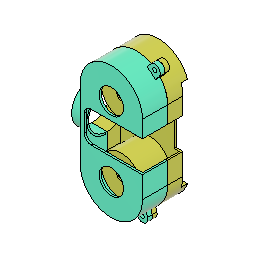
Nerf Ultra 2 cage v5 (Autodesk Fusion 360 design; units mm, degrees)
Autodesk Fusion 360 part; units mm, degrees
note: some values were not read from the file. Set by a fixed rule: which sketch regions a step uses.
sketch "Sketch1" plane through (0, 0, 0) normal (0, 0, 1) x (1, 0, 0)
  line L0 (23, 48.75) -> (-23, 48.75)
  line L1 (-23, 48.75) -> (-23, -48.75)
  line L2 (-23, -48.75) -> (23, -48.75)
  line L3 (23, -48.75) -> (23, 48.75)
  line L4 (23, 48.75) -> (-23, -48.75) construction
  line L5 (-23, 48.75) -> (23, -48.75) construction
  arc A0 (23, 25.75) -> (-23, 25.75) centre (0, 25.75) ccw
  arc A1 (-23, -25.75) -> (23, -25.75) centre (0, -25.75) ccw
  dimension "d1" = 46
  dimension "d2" = 97.5
  constraint perpendicular L0 L1
  constraint parallel L0 L2
  constraint parallel L1 L3
  constraint horizontal L0
  constraint coincident L4 origin
  constraint coincident L5 origin
  constraint tangent L3 A0
  constraint coincident L3 A0.start
  constraint coincident L1 A0.end
  constraint tangent L0 A0
  constraint tangent L1 A0
  constraint coincident L3 A1.end
  constraint coincident L1 A1.start
  constraint tangent L2 A1
  constraint tangent L3 A1
  constraint tangent L1 A1
  measures "d1" distance of L1.end L2.end
  measures "d2" distance of L0.end L1.end
  measures "d34" distance of L0.start
  measures "d93" diameter of L0.start
extrude "Extrude1" add sketch "Sketch1" along normal blind 16 contours L1 L3 A0 A1 makes body 1
sketch "Sketch2" plane through (0, 0, 16) normal (0, 0, 1) x (1, 0, 0)
  arc A0 (-23, -25.75) -> (23, -25.75) centre (0, -25.75) ccw
  line L0 (23, -25.75) -> (23, 25.75)
  arc A1 (23, 25.75) -> (-23, 25.75) centre (0, 25.75) ccw
  line L1 (-23, 25.75) -> (-23, -25.75)
  line L2 (0, 0) -> (-28, 0) construction
  line L3 (-23, 25) -> (-33, 25)
  line L4 (-33, 25) -> (-33, -25)
  line L5 (-33, -25) -> (-23, -25)
  line L6 (-23, -25) -> (-23, 25)
  line L7 (-23, 25) -> (-33, -25) construction
  line L8 (-33, 25) -> (-23, -25) construction
  circle A2 centre (-28, 18) radius 2.5
  circle A3 centre (-28, 18) radius 1.5
  circle A4 centre (-28, -18) radius 2.5
  circle A5 centre (-28, -18) radius 1.5
  line L9 (-28, -18) -> (-28, 18) construction
  point P0 (-28, 0)
  point P1 (-23, 0)
  dimension "d5" = 50
  dimension "d6" = 10
  dimension "d7" = 36
  dimension "d8" = 5
  dimension "d9" = 3
  constraint coincident L2.start origin
  constraint perpendicular L1 L2
  constraint perpendicular L3 L4
  constraint parallel L3 L5
  constraint parallel L4 L6
  constraint horizontal L3
  constraint coincident L7 P0
  constraint coincident L8 P0
  constraint coincident P0 L2.end
  constraint midpoint L6 P1
  constraint coincident L1 P1
  constraint concentric A2 A3
  constraint concentric A4 A5
  constraint equal A2 A4
  constraint equal A3 A5
  constraint coincident A4.centre A5.centre
  constraint coincident A2.centre A3.centre
  constraint vertical L9
  constraint midpoint P0 L9
  measures "d5" distance of L3.start L5.end
  measures "d6" distance of L3.start L3.end
  measures "d7" distance of A4.centre A2.centre
  measures "d8" diameter of A2
  measures "d9" diameter of A3
extrude "Extrude2" add sketch "Sketch2" against normal blind 1.3 contours L1 L3 L4 L5 L6 bodies 1
extrude "Extrude3" add sketch "Sketch2" along normal blind 1 and the other way blind 1.3 contours A2 | A4 bodies 1
sketch "Sketch3" plane through (0, 0, 14.7) normal (0, 0, -1) x (-1, 0, 0)
  circle A0 centre (28, -18) radius 1.5
  circle A1 centre (28, 18) radius 1.5
  line L0 (23, 25) -> (23, -25)
  line L1 (23, -25) -> (33, -25)
  line L2 (33, -25) -> (33, 25)
  line L3 (33, 25) -> (23, 25)
  circle A2 centre (28, 18) radius 4
  circle A3 centre (28, -18) radius 4
  circle A4 centre (28, 18) radius 2.7
  circle A5 centre (28, -18) radius 2.7
  dimension "d16" = 8
  dimension "d17" = 5.4
  constraint concentric A1 A2
  constraint concentric A0 A3
  constraint equal A2 A3
  constraint concentric A2 A4
  constraint concentric A0 A5
  constraint equal A4 A5
  measures "d16" diameter of A2
  measures "d17" diameter of A4
extrude "Extrude4" add sketch "Sketch3" along normal blind 2.25 contours A2 | A3 bodies 1
sketch "Sketch5" plane through (0, 0, 16) normal (0, 0, 1) x (1, 0, 0)
  circle A0 centre (-28, 18) radius 2.5
  circle A1 centre (-28, -18) radius 2.5
  arc A2 (-23, -25.75) -> (23, -25.75) centre (0, -25.75) ccw
  line L0 (23, -25.75) -> (23, 25.75)
  arc A3 (23, 25.75) -> (-23, 25.75) centre (0, 25.75) ccw
  line L1 (-23, 25.75) -> (-23, 25)
  line L2 (-23, 25) -> (-33, 25)
  line L3 (-33, 25) -> (-33, -25)
  line L4 (-33, -25) -> (-23, -25)
  line L5 (-23, -25) -> (-23, -25.75)
  line L6 (23, 13.25) -> (18, 13.25)
  line L7 (18, 13.25) -> (18, -9.75)
  line L8 (18, -9.75) -> (23, -9.75)
  line L9 (23, -9.75) -> (23, 13.25)
  line L10 (23, 13.25) -> (18, -9.75) construction
  line L11 (18, 13.25) -> (23, -9.75) construction
  point P0 (20.5, 1.75)
  point P1 (0, -48.75)
  dimension "d27" = 23
  dimension "d28" = 5
  dimension "d34" = 39
  constraint perpendicular L6 L7
  constraint parallel L6 L8
  constraint parallel L7 L9
  constraint horizontal L6
  constraint coincident L0 L6.start
  constraint coincident L10 P0
  constraint coincident L11 P0
  constraint midpoint A2 P1
  measures "d27" distance of L6 L8
  measures "d28" distance of L6.start L6.end
  measures "d34" vertical distance of L7.end P1
extrude "Extrude5" cut sketch "Sketch5" against normal blind 20 contours L0 L6 L7 L8 L9 bodies 1
sketch "Sketch8" plane through (0, 0, 16) normal (0, 0, 1) x (1, 0, 0)
  line L0 (18, 13.25) -> (23, 13.25)
  line L1 (23, 13.25) -> (23, 25.75)
  arc A0 (23, 25.75) -> (-23, 25.75) centre (0, 25.75) ccw
  line L2 (-23, 25.75) -> (-23, 25)
  line L3 (-23, 25) -> (-33, 25)
  line L4 (-33, 25) -> (-33, -25)
  line L5 (-33, -25) -> (-23, -25)
  line L6 (-23, -25) -> (-23, -25.75)
  arc A1 (-23, -25.75) -> (23, -25.75) centre (0, -25.75) ccw
  line L7 (23, -25.75) -> (23, -9.75)
  line L8 (23, -9.75) -> (18, -9.75)
  line L9 (18, -9.75) -> (18, 13.25) construction
  circle A2 centre (-28, 18) radius 2.5
  circle A3 centre (-28, -18) radius 2.5
  line L10 (16.7, -11.05) -> (16.7, 14.55) construction
  line L11 (16.7, 14.55) -> (21.7, 14.55)
  line L12 (21.7, 14.55) -> (21.7, 25.75)
  arc A4 (21.7, 25.75) -> (-21.7, 25.75) centre (0, 25.75) ccw
  line L13 (-21.7, 25.75) -> (-21.7, 23.7)
  line L14 (-21.7, 23.7) -> (-31.7, 23.7)
  line L15 (-31.7, 23.7) -> (-31.7, -23.7)
  line L16 (-31.7, -23.7) -> (-21.7, -23.7)
  line L17 (-21.7, -23.7) -> (-21.7, -25.75)
  arc A5 (-21.7, -25.75) -> (21.7, -25.75) centre (0, -25.75) ccw
  line L18 (21.7, -25.75) -> (21.7, -11.05)
  line L19 (21.7, -11.05) -> (16.7, -11.05)
  line L20 (21.7, -11.05) -> (21.7, 14.55)
  line L21 (-21.7, 23.7) -> (-21.7, -23.7)
  dimension "d52" = -1.3
extrude "Extrude11" cut sketch "Sketch8" against normal blind 9.9 contours L12 A4 L13 L17 A5 L18 L20 L21 bodies 1
delete_face "DeleteFace1" 1 faces at (-21.7, 7.9, 12.7) on bodies 1
delete_face "DeleteFace2" 1 faces at (-21.7, -25.0652, 12.7) on bodies 1
sketch "Sketch4" plane through (0, 0, 16) normal (0, 0, 1) x (1, 0, 0)
  circle A0 centre (-28, 18) radius 2.5
  circle A1 centre (-28, -18) radius 2.5
  arc A2 (-23, -25.75) -> (23, -25.75) centre (0, -25.75) ccw
  line L0 (23, 13.25) -> (23, 25.75)
  arc A3 (23, 25.75) -> (-23, 25.75) centre (0, 25.75) ccw
  line L1 (-23, 25.75) -> (-23, 25)
  line L2 (-23, 25) -> (-33, 25)
  line L3 (-33, 25) -> (-33, -25)
  line L4 (-33, -25) -> (-23, -25)
  line L5 (-23, -25) -> (-23, -25.75)
  line L6 (11.2138, 45.8311) -> (17.4138, 40.7753)
  line L7 (17.4138, 40.7753) -> (22.6279, 47.1694)
  line L8 (22.6279, 47.1694) -> (16.4279, 52.2252) construction
  line L9 (16.4279, 52.2252) -> (11.2138, 45.8311)
  line L10 (2.696, -48.5914) -> (10.3567, -46.2863)
  line L11 (10.3567, -46.2863) -> (12.734, -54.1869)
  line L12 (12.734, -54.1869) -> (5.0733, -56.492) construction
  line L13 (5.0733, -56.492) -> (2.696, -48.5914)
  arc A4 (3.9208, -52.6617) -> (11.5814, -50.3565) centre (7.7511, -51.5091) ccw
  arc A5 (20.1, 44.0694) -> (13.9, 49.1252) centre (17, 46.5973) ccw
  line L14 (8.9037, -55.3394) -> (6.6273, -47.7745) construction
  line L15 (19.5279, 49.6973) -> (14.5353, 43.5748) construction
  circle A6 centre (17, 46.5973) radius 2.7
  circle A7 centre (7.7511, -51.5091) radius 2.7
  circle A8 centre (7.7511, -51.5091) radius 2.5
  circle A9 centre (17, 46.5973) radius 2.5
  line L16 (21.7, 13.25) -> (23, 13.25)
  line L17 (23, -25.75) -> (23, -9.75)
  line L18 (23, -9.75) -> (21.7, -9.75)
  circle A10 centre (7.7511, -51.5091) radius 1.5
  circle A11 centre (17, 46.5973) radius 1.5
  line L19 (21.7, -9.75) -> (21.7, -25.75)
  arc A12 (-21.7, -25.75) -> (21.7, -25.75) centre (0, -25.75) ccw
  line L20 (-21.7, -25.75) -> (-21.7, 25.75)
  arc A13 (21.7, 25.75) -> (-21.7, 25.75) centre (0, 25.75) ccw
  line L21 (21.7, 25.75) -> (21.7, 13.25)
  dimension "d20" = 8
  dimension "d21" = 7.9
  dimension "d22" = 5.4
  dimension "d23" = 5.4
  dimension "d24" = 5
  dimension "d25" = 5
  dimension "d38" = 3
  dimension "d39" = 3
  dimension "d59" = 49
  dimension "d63" = 45
  constraint perpendicular L6 L7
  constraint parallel L6 L8
  constraint parallel L7 L9
  constraint coincident A3 L6.end
  constraint coincident A3 L6.start
  constraint perpendicular L10 L11
  constraint parallel L10 L12
  constraint parallel L11 L13
  constraint coincident A2 L10.end
  constraint coincident A2 L10.start
  constraint coincident L11 A4.end
  constraint coincident L13 A4.start
  constraint tangent L9 A5
  constraint coincident L7 A5.start
  constraint coincident L9 A5.end
  constraint tangent L8 A5
  constraint tangent L7 A5
  constraint tangent L13 A4
  constraint tangent L11 A4
  constraint equal L7 L13
  constraint equal L8 L12
  constraint tangent L12 A4
  constraint midpoint L12 L14.start
  constraint coincident A2 L14.end
  constraint perpendicular L10 L14
  constraint midpoint L8 L15.start
  constraint coincident A3 L15.end
  constraint perpendicular L8 L15
  constraint concentric A5 A6
  constraint concentric A4 A7
  constraint concentric A7 A8
  constraint concentric A5 A9
  constraint concentric A8 A10
  constraint concentric A5 A11
  measures "d20" distance of L11.end L12.end
  measures "d21" distance of L14.start L14.end
  measures "d22" diameter of A6
  measures "d23" diameter of A7
  measures "d24" diameter of A8
  measures "d25" diameter of A9
  measures "d38" diameter of A10
  measures "d39" diameter of A11
  measures "d59" distance of A1.centre A4.centre
  measures "d63" horizontal distance of A0.centre A5.centre
extrude "Extrude6" add sketch "Sketch4" against normal blind 3.5 contours A2 L11 L13 A4 | A3 L7 L9 A5 | A6 | A7 bodies 1
extrude "Extrude7" add sketch "Sketch4" along normal blind 1 and the other way blind 0.9 contours A8 | A9 bodies 1
sketch "Sketch7" plane through (-33, 0, 0) normal (-1, 0, 0) x (0, 0, 1)
  line L0 (16, -25) -> (16, 25)
  line L1 (16, 25) -> (14.7, 25)
  line L2 (14.7, 25) -> (14.7, -25)
  line L3 (14.7, -25) -> (16, -25)
  circle A0 centre (16, 0) radius 13.75
  circle A1 centre (16, 0) radius 15.05
  point P0 (17, -18)
  dimension "d46" = 27.5
  dimension "d47" = 30.1
  dimension "d74" = 18
  constraint concentric A0 A1
  constraint coincident L0 A0.centre
  measures "d46" diameter of A0
  measures "d47" diameter of A1
  measures "d74" vertical distance of A0.centre P0
extrude "Extrude9" cut sketch "Sketch7" against normal blind 11.3 contours L0 L2 A0 | L0 A0 | L2 A0 bodies 1
extrude "Extrude10" add sketch "Sketch7" against normal blind 10 contours L2 A0 A1 bodies 1
ref_plane "WorkPlane1" through (-5, -2.12, 36) normal (0, 0, 1) x (1, 0, 0)
sketch "Sketch10" plane through (-4.5034, 32.8919, 36) normal (0, 0, 1) x (1, 0, 0)
  line L0 (27.5034, -19.6419) -> (27.5034, -7.1419)
  arc A0 (27.5034, -7.1419) -> (21.9172, 7.8834) centre (4.5034, -7.1419) ccw
  line L1 (21.9172, 7.8834) -> (24.6034, 11.1775)
  arc A1 (24.6034, 11.1775) -> (18.4034, 16.2332) centre (21.5034, 13.7054) ccw
  line L2 (18.4034, 16.2332) -> (15.7172, 12.9391)
  arc A2 (15.7172, 12.9391) -> (-18.4966, -7.1419) centre (4.5034, -7.1419) ccw
  line L3 (-18.4966, -7.1419) -> (-18.4966, -7.8919)
  line L4 (-18.4966, -7.8919) -> (-28.4966, -7.8919)
  line L5 (-28.4966, -7.8919) -> (-28.4966, -19.1419)
  circle A3 centre (21.5034, 13.7054) radius 2.5
  circle A4 centre (-23.4966, -14.8919) radius 2.5
  line L6 (-28.4966, -46.6419) -> (-28.4966, -57.8919)
  line L7 (-28.4966, -57.8919) -> (-18.4966, -57.8919)
  line L8 (-18.4966, -57.8919) -> (-18.4966, -58.6419)
  arc A5 (-18.4966, -58.6419) -> (7.1994, -81.4834) centre (4.5034, -58.6419) ccw
  line L9 (7.1994, -81.4834) -> (8.4241, -85.5536)
  arc A6 (8.4241, -85.5536) -> (16.0848, -83.2484) centre (12.2545, -84.401) ccw
  line L10 (16.0848, -83.2484) -> (14.8601, -79.1782)
  arc A7 (14.8601, -79.1782) -> (27.5034, -58.6419) centre (4.5034, -58.6419) ccw
  line L11 (27.5034, -58.6419) -> (27.5034, -42.6419)
  circle A8 centre (-23.4966, -50.8919) radius 2.5
  circle A9 centre (12.2545, -84.401) radius 2.5
  line L12 (-28.4966, -46.6419) -> (-28.4966, -19.1419)
  line L13 (27.5034, -42.6419) -> (27.5034, -19.6419)
  line L14 (-17.1966, -58.6419) -> (-17.1966, -46.6419)
  constraint coincident L6.start L12.start
  constraint coincident L5.end L12.end
  constraint coincident L11.end L13.start
  constraint coincident L0.start L13.end
extrude "Extrude12" add sketch "Sketch10" along normal blind 0.6 separate body makes body 2
sketch "Sketch11" plane through (0, 0, 0) normal (0, 0, -1) x (-1, 0, 0)
  line L0 (-23, 13.25) -> (-18, 13.25)
  line L1 (-18, 13.25) -> (-18, -9.75)
  line L2 (-18, -9.75) -> (-23, -9.75)
  line L3 (-23, -9.75) -> (-23, -25.75)
  arc A0 (-23, -25.75) -> (23, -25.75) centre (0, -25.75) ccw
  line L4 (23, -25.75) -> (23, 25.75)
  arc A1 (23, 25.75) -> (-23, 25.75) centre (0, 25.75) ccw
  line L5 (-23, 25.75) -> (-23, 13.25)
  circle A2 centre (0, 25.75) radius 14.8
  circle A3 centre (0, -25.75) radius 14.8
  dimension "d66" = 29.6
  constraint concentric A1 A2
  constraint concentric A0 A3
  constraint equal A2 A3
  measures "d66" diameter of A2
extrude "Extrude13" add sketch "Sketch11" against normal blind 27.35 contours A2 | A3 bodies 1
sketch "Sketch9" plane through (0, 0, 0) normal (0, 0, -1) x (-1, 0, 0)
  line L0 (-23, 13.25) -> (-18, 13.25)
  line L1 (-18, 13.25) -> (-18, -9.75)
  line L2 (-18, -9.75) -> (-23, -9.75)
  line L3 (-23, -9.75) -> (-23, -25.75)
  arc A0 (-23, -25.75) -> (23, -25.75) centre (0, -25.75) ccw
  line L4 (23, -25.75) -> (23, 25.75)
  arc A1 (23, 25.75) -> (-23, 25.75) centre (0, 25.75) ccw
  line L5 (6.7, 20.15) -> (23, 20.15)
  line L6 (23, 20.15) -> (23, -20.15)
  line L7 (23, -20.15) -> (6.7, -20.15)
  line L8 (6.7, -20.15) -> (6.7, 20.15)
  circle A2 centre (0, 25.75) radius 13.65
  circle A3 centre (0, -25.75) radius 13.65
  line L9 (-23, 25.75) -> (-23, 13.25)
  line L10 (6.7, 7.6) -> (-5, 7.6)
  line L11 (-5, 7.6) -> (-5, -7.6)
  line L12 (-5, -7.6) -> (6.7, -7.6)
  line L13 (6.7, -7.6) -> (6.7, 7.6)
  line L14 (31.1452, 33.45) -> (-33.5103, 33.45)
  line L15 (-33.5103, 33.45) -> (-33.5103, 56.976)
  line L16 (-33.5103, 56.976) -> (31.1452, 56.976)
  line L17 (31.1452, 56.976) -> (31.1452, 33.45)
  line L18 (-33.5103, -63.22) -> (26.4357, -63.22)
  line L19 (26.4357, -63.22) -> (26.4357, -33.45)
  line L20 (26.4357, -33.45) -> (-33.5103, -33.45)
  line L21 (-33.5103, -33.45) -> (-33.5103, -63.22)
  dimension "d55" = 40.3
  dimension "d56" = 27.3
  dimension "d67" = 16.3
  dimension "d68" = 15.2
  dimension "d69" = 28
  dimension "d70" = 13.3
  dimension "d71" = 13.3
  constraint horizontal L5
  constraint vertical L6
  constraint horizontal L7
  constraint vertical L8
  constraint concentric A1 A2
  constraint concentric A0 A3
  constraint midpoint L4 L6
  constraint equal A2 A3
  constraint horizontal L10
  constraint vertical L11
  constraint horizontal L12
  constraint vertical L13
  constraint coincident L8 L10.start
  constraint midpoint L8 L13
  constraint horizontal L14
  constraint vertical L15
  constraint horizontal L16
  constraint vertical L17
  constraint horizontal L18
  constraint vertical L19
  constraint horizontal L20
  constraint vertical L21
  measures "d55" distance of L5.start L7.end
  measures "d56" diameter of A2
  measures "d67" distance of L6 L8
  measures "d68" distance of L10 L12
  measures "d69" distance of L6 L11
  measures "d70" distance of L7 L20
  measures "d71" distance of L5 L14
extrude "Extrude14" cut sketch "Sketch9" against normal blind 26.5 contours L5 L8 A2 L14 | A2 L14 | L5 L8 A2 | A3 L20 | L7 L8 A3 L20 | L7 L8 A3 bodies 1
extrude "Extrude15" cut sketch "Sketch9" against normal blind 4.7 contours L0 L1 L2 L3 A0 A1 L8 A2 A3 L9 L10 L11 L12 L14 L20 | L4 A1 L5 A2 L14 | A0 L4 L7 A3 L20 bodies 1
sketch "Sketch12" plane through (0, 0, 27.35) normal (0, 0, 1) x (1, 0, 0)
  circle A0 centre (0, -25.75) radius 14.8
  circle A1 centre (0, -25.75) radius 3.225
  circle A2 centre (0, 25.75) radius 3.225
  circle A3 centre (0, 25.75) radius 14.8
  dimension "d77" = 6.45
  constraint concentric A0 A1
  constraint equal A1 A2
  constraint concentric A2 A3
  measures "d77" diameter of A1
extrude "Extrude16" cut sketch "Sketch12" against normal through all contours A1 | A2 bodies 1
sketch "Sketch13" plane through (0, 0, 4.7) normal (0, 0, -1) x (-1, 0, 0)
  line L0 (12.4484, 20.15) -> (23, 20.15)
  line L1 (23, 20.15) -> (23, 25.75)
  arc A0 (23, 25.75) -> (21.6728, 33.45) centre (0, 25.75) ccw
  line L2 (21.6728, 33.45) -> (11.2709, 33.45)
  arc A1 (12.4484, 20.15) -> (11.2709, 33.45) centre (0, 25.75) ccw
  circle A2 centre (0, 25.75) radius 14.8
  circle A3 centre (0, -25.75) radius 14.8
  circle A4 centre (0, 25.75) radius 14.8
  circle A5 centre (0, -25.75) radius 14.8
  line L3 (21.7, -9.5421) -> (21.7, -25.75)
  arc A6 (-21.7, -25.75) -> (21.7, -25.75) centre (0, -25.75) ccw
  line L4 (-21.7, -25.75) -> (-21.7, -9.75)
  line L5 (-21.7, -9.75) -> (-18, -9.75)
  line L6 (-18, -9.75) -> (-18, 13.25)
  line L7 (-18, 13.25) -> (-21.7, 13.25)
  line L8 (-21.7, 13.25) -> (-21.7, 25.75)
  arc A7 (21.7, 25.75) -> (-21.7, 25.75) centre (0, 25.75) ccw
  line L9 (21.7, 25.75) -> (21.7, 9.5421)
  line L10 (21.7, 9.5421) -> (21.7, -9.5421)
  circle A8 centre (18.25, 25.75) radius 2
  circle A9 centre (-18.25, 25.75) radius 2
  circle A10 centre (-18.25, -25.75) radius 2
  circle A11 centre (18.25, -25.75) radius 2
  line L11 (-21.7, 25.75) -> (-14.8, 25.75) construction
  line L12 (-14.8, 25.75) -> (14.8, 25.75) construction
  line L13 (14.8, 25.75) -> (21.7, 25.75) construction
  line L14 (-21.7, -25.75) -> (-14.8, -25.75) construction
  line L15 (-14.8, -25.75) -> (14.8, -25.75) construction
  line L16 (14.8, -25.75) -> (21.7, -25.75) construction
  dimension "d79" = 4
  constraint equal A8 A11
  constraint equal A8 A9
  constraint equal A9 A10
  constraint coincident L8.end A7.end
  constraint coincident A2 L11.end
  constraint coincident A4 L12.end
  constraint coincident A7.start L9.start
  constraint coincident A6.start L4.start
  constraint coincident A5 L14.end
  constraint coincident A3 L15.end
  constraint coincident L3.end A6.end
  constraint midpoint A11.centre L16
  constraint midpoint A10.centre L14
  constraint midpoint A9.centre L11
  constraint midpoint A8.centre L13
  constraint midpoint A0.centre L12
  constraint midpoint A3.centre L15
  constraint horizontal L15
  constraint horizontal L12
  measures "d79" diameter of A8
extrude "Extrude17" cut sketch "Sketch13" against normal through all contours A8 | A9 | A10 | A11 bodies 1
sketch "Sketch14" plane through (0, 0, 16) normal (0, 0, 1) x (1, 0, 0)
  line L0 (-33, 13.75) -> (-21.7, 13.75)
  line L1 (-21.7, 13.75) -> (-21.7, 25.75)
  arc A0 (21.7, 25.75) -> (-21.7, 25.75) centre (0, 25.75) ccw
  line L2 (21.7, 25.75) -> (21.7, 13.25)
  line L3 (21.7, 13.25) -> (23, 13.25)
  line L4 (23, 13.25) -> (23, 25.75)
  arc A1 (23, 25.75) -> (17.4138, 40.7753) centre (0, 25.75) ccw
  line L5 (17.4138, 40.7753) -> (20.1, 44.0694)
  arc A2 (20.1, 44.0694) -> (13.9, 49.1252) centre (17, 46.5973) ccw
  line L6 (13.9, 49.1252) -> (11.2138, 45.8311)
  arc A3 (11.2138, 45.8311) -> (-23, 25.75) centre (0, 25.75) ccw
  line L7 (-23, 25.75) -> (-23, 25)
  line L8 (-23, 25) -> (-33, 25)
  line L9 (-33, 25) -> (-33, 13.75)
  circle A4 centre (17, 46.5973) radius 2.5
  circle A5 centre (-28, 18) radius 2.5
  circle A6 centre (-28, -18) radius 2.5
  line L10 (-21.7, -13.75) -> (-33, -13.75)
  line L11 (-33, -13.75) -> (-33, -25)
  line L12 (-33, -25) -> (-23, -25)
  line L13 (-23, -25) -> (-23, -25.75)
  arc A7 (-23, -25.75) -> (2.696, -48.5914) centre (0, -25.75) ccw
  line L14 (2.696, -48.5914) -> (3.9208, -52.6617)
  arc A8 (3.9208, -52.6617) -> (11.5814, -50.3565) centre (7.7511, -51.5091) ccw
  line L15 (11.5814, -50.3565) -> (10.3567, -46.2863)
  arc A9 (10.3567, -46.2863) -> (23, -25.75) centre (0, -25.75) ccw
  line L16 (23, -25.75) -> (23, -9.75)
  line L17 (23, -9.75) -> (21.7, -9.75)
  line L18 (21.7, -9.75) -> (21.7, -25.75)
  arc A10 (-21.7, -25.75) -> (21.7, -25.75) centre (0, -25.75) ccw
  line L19 (-21.7, -25.75) -> (-21.7, -13.75)
  circle A11 centre (7.7511, -51.5091) radius 2.5
extrude "Extrude1'" add sketch "Sketch14" along normal blind 1.25 separate body makes body 3 at (-28.0623, 23.4977, 16) makes body 4 at (-27.9377, -23.4977, 16) in component "Component"
sketch "Sketch15" plane through (0, 0, 17.25) normal (0, 0, 1) x (1, 0, 0)
  circle A0 centre (7.7511, -51.5091) radius 2.5
  circle A1 centre (-28, -18) radius 2.5
  line L0 (-21.7, -25.75) -> (-21.7, -13.75)
  line L1 (-21.7, -13.75) -> (-33, -13.75)
  line L2 (-33, -13.75) -> (-33, -25)
  line L3 (-33, -25) -> (-23, -25)
  line L4 (-23, -25) -> (-23, -25.75)
  arc A2 (-23, -25.75) -> (2.696, -48.5914) centre (0, -25.75) ccw
  line L5 (2.696, -48.5914) -> (3.9208, -52.6617)
  arc A3 (3.9208, -52.6617) -> (11.5814, -50.3565) centre (7.7511, -51.5091) ccw
  line L6 (11.5814, -50.3565) -> (10.3567, -46.2863)
  arc A4 (10.3567, -46.2863) -> (23, -25.75) centre (0, -25.75) ccw
  line L7 (23, -25.75) -> (23, -9.75)
  line L8 (23, -9.75) -> (21.7, -9.75)
  line L9 (21.7, -9.75) -> (21.7, -25.75)
  arc A5 (-21.7, -25.75) -> (21.7, -25.75) centre (0, -25.75) ccw
  circle A6 centre (17, 46.5973) radius 2.5
  circle A7 centre (-28, 18) radius 2.5
  line L10 (21.7, 25.75) -> (21.7, 13.25)
  line L11 (21.7, 13.25) -> (23, 13.25)
  line L12 (23, 13.25) -> (23, 25.75)
  arc A8 (23, 25.75) -> (17.4138, 40.7753) centre (0, 25.75) ccw
  line L13 (17.4138, 40.7753) -> (20.1, 44.0694)
  arc A9 (20.1, 44.0694) -> (13.9, 49.1252) centre (17, 46.5973) ccw
  line L14 (13.9, 49.1252) -> (11.2138, 45.8311)
  arc A10 (11.2138, 45.8311) -> (-23, 25.75) centre (0, 25.75) ccw
  line L15 (-23, 25.75) -> (-23, 25)
  line L16 (-23, 25) -> (-33, 25)
  line L17 (-33, 25) -> (-33, 13.75)
  line L18 (-33, 13.75) -> (-21.7, 13.75)
  line L19 (-21.7, 13.75) -> (-21.7, 25.75)
  arc A11 (21.7, 25.75) -> (-21.7, 25.75) centre (0, 25.75) ccw
  line L20 (-23, 25) -> (-23, -25)
  circle A12 centre (0, -25.75) radius 23
  circle A13 centre (0, 25.75) radius 23
  constraint coincident L15.end L16.start
  constraint coincident L3.end L4.start
  constraint concentric A2 A12
  constraint coincident L6.end A12
  constraint concentric A8 A13
  constraint coincident A8.end A13
extrude "Extrude2'" add sketch "Sketch15" along normal blind 17.4 contours L0 A2 A4 L9 A5 A12 | L0 L1 L4 L20 A12 | L7 L8 L9 A12 | L10 A8 A10 L19 A11 A13 | L10 L11 L12 A13 | L15 L18 L19 L20 A13 bodies 3 4 in component "Component"
sketch "Sketch16" plane through (-33, 0, 0) normal (-1, 0, 0) x (0, 0, 1)
  line L0 (16, -13.75) -> (16, -25)
  line L1 (16, -25) -> (17.25, -25)
  line L2 (17.25, -25) -> (17.25, -13.75)
  line L3 (17.25, -13.75) -> (16, -13.75)
  arc A0 (16, 13.75) -> (16, -13.75) centre (16, 0) ccw
  arc A1 (14.7, 14.9937) -> (14.7, -14.9937) centre (16, 0) ccw
  circle A2 centre (16, 0) radius 13.75
  circle A3 centre (16, 0) radius 15.05
  line L4 (16, 13.75) -> (16, 15.05)
  line L5 (16, -13.75) -> (16, -15.05)
  constraint concentric A1 A2
  constraint coincident A0.start A2
  constraint concentric A2 A3
  constraint coincident A1.start A3
  constraint coincident A0.start L4.start
  constraint coincident A3 L4.end
  constraint vertical L4
  constraint coincident L0.start L3.end
  constraint coincident A3 L5.end
  constraint coincident L0 L5.end
extrude "Extrude3'" add sketch "Sketch16" against normal blind 11.3 contours L2 L3 A2 A3 L4 bodies 3 4 in component "Component"
sketch "Sketch17" plane through (0, 0, 34.65) normal (0, 0, 1) x (1, 0, 0)
  line L0 (21.7, 25.75) -> (21.7, 13.25)
  line L1 (21.7, 13.25) -> (23, 13.25)
  line L2 (23, 13.25) -> (23, 25.75)
  arc A0 (23, 25.75) -> (-23, 25.75) centre (0, 25.75) ccw
  line L3 (-23, 25.75) -> (-23, 25)
  line L4 (-23, 25) -> (-23, 13.75)
  line L5 (-23, 13.75) -> (-21.7, 13.75)
  line L6 (-21.7, 13.75) -> (-21.7, 25.75)
  arc A1 (21.7, 25.75) -> (-21.7, 25.75) centre (0, 25.75) ccw
  line L7 (-21.7, -25.75) -> (-21.7, -13.75)
  line L8 (-21.7, -13.75) -> (-23, -13.75)
  line L9 (-23, -13.75) -> (-23, -25)
  line L10 (-23, -25) -> (-23, -25.75)
  arc A2 (-23, -25.75) -> (23, -25.75) centre (0, -25.75) ccw
  line L11 (23, -25.75) -> (23, -9.75)
  line L12 (23, -9.75) -> (21.7, -9.75)
  line L13 (21.7, -9.75) -> (21.7, -25.75)
  arc A3 (-21.7, -25.75) -> (21.7, -25.75) centre (0, -25.75) ccw
  line L14 (-23, -13.75) -> (-23, 13.75)
  line L15 (-21.7, 13.75) -> (-21.7, -13.75)
  constraint coincident L8.end L9.start
  constraint coincident L4.end L5.start
  constraint coincident L5.end L6.start
  constraint coincident L7.end L8.start
extrude "Extrude4'" add sketch "Sketch17" along normal up to surface contours L5 L8 L14 L15 end surface at (-29.2333, 12.5046, 24.3747) on bodies 3 bodies 3 in component "Component"
sketch "Sketch18" plane through (0, 0, 17.25) normal (0, 0, 1) x (1, 0, 0)
  circle A0 centre (-28, 18) radius 2.5
  line L0 (-33, 14.998) -> (-23, 14.998)
  line L1 (-23, 14.998) -> (-23, 25)
  line L2 (-23, 25) -> (-33, 25)
  line L3 (-33, 25) -> (-33, 14.998)
  circle A1 centre (-28, 18) radius 3.95
  line L4 (-23, -14.998) -> (-33, -14.998)
  line L5 (-33, -14.998) -> (-33, -25)
  line L6 (-33, -25) -> (-23, -25)
  line L7 (-23, -25) -> (-23, -14.998)
  circle A2 centre (-28, -18) radius 2.5
  circle A3 centre (-28, -18) radius 3.95
  dimension "d89" = 7.9
  dimension "d90" = 7.9
  constraint concentric A0 A1
  constraint concentric A2 A3
  measures "d89" diameter of A1
  measures "d90" diameter of A3
extrude "Extrude5'" add sketch "Sketch18" along normal blind 2.3 contours L0 A1 | L0 A1 | L4 A3 | L4 A3 bodies 3 in component "Component"
sketch "Sketch19" plane through (0, 0, 34.65) normal (0, 0, 1) x (1, 0, 0)
  line L0 (21.7, 25.75) -> (21.7, 13.25)
  line L1 (21.7, 13.25) -> (23, 13.25)
  line L2 (23, 13.25) -> (23, 25.75)
  arc A0 (23, 25.75) -> (-23, 25.75) centre (0, 25.75) ccw
  line L3 (-23, 25.75) -> (-23, 25)
  line L4 (-23, 25) -> (-23, -25)
  line L5 (-23, -25) -> (-23, -25.75)
  arc A1 (-23, -25.75) -> (23, -25.75) centre (0, -25.75) ccw
  line L6 (23, -25.75) -> (23, -9.75)
  line L7 (23, -9.75) -> (21.7, -9.75)
  line L8 (21.7, -9.75) -> (21.7, -25.75)
  arc A2 (-21.7, -25.75) -> (21.7, -25.75) centre (0, -25.75) ccw
  line L9 (-21.7, -25.75) -> (-21.7, 13.75)
  line L10 (-21.7, 13.75) -> (-21.7, 25.75)
  arc A3 (21.7, 25.75) -> (-21.7, 25.75) centre (0, 25.75) ccw
  circle A4 centre (0, -25.75) radius 9
  circle A5 centre (0, 25.75) radius 9
  line L11 (21.7, 13.25) -> (21.7, -9.75)
  line L12 (21.7, -9.75) -> (-15, -9.75)
  line L13 (-21.7, -9.75) -> (-21.7, 13.25)
  line L14 (-15, 13.25) -> (21.7, 13.25)
  line L15 (-20, 8.25) -> (-20, -4.75)
  arc A6 (-15, 13.25) -> (-20, 8.25) centre (-15, 8.25) ccw
  arc A7 (-20, -4.75) -> (-15, -9.75) centre (-15, -4.75) ccw
  dimension "d93" = 18
  dimension "d94" = 18
  dimension "d95" = 3
  dimension "d96" = 5
  dimension "d97" = 5
  constraint concentric A1 A4
  constraint concentric A0 A5
  constraint perpendicular L11 L12
  constraint parallel L11 L13
  constraint parallel L12 L14
  constraint coincident L7.end L8.start
  constraint perpendicular L7 L11
  constraint coincident L0.end L1.start
  constraint perpendicular L12 L15
  constraint coincident L13.end L14
  constraint tangent L15 A6
  constraint tangent L14 A6
  constraint coincident L13.start L12
  constraint tangent L15 A7
  constraint tangent L12 A7
  measures "d93" diameter of A4
  measures "d94" diameter of A5
  measures "d95" distance of L4 L15
  measures "d96" radius of A6
  measures "d97" radius of A7
extrude "Extrude6'" add sketch "Sketch19" against normal blind 1.5 contours L0 L8 A2 L9 L10 A3 L12 L13 L14 L15 A6 A7 bodies 3 in component "Component"
sketch "Sketch20" plane through (0, 0, 17.25) normal (0, 0, 1) x (1, 0, 0)
  arc A0 (2.696, -48.5914) -> (10.3567, -46.2863) centre (0, -25.75) ccw
  line L0 (2.696, -48.5914) -> (3.9208, -52.6617)
  arc A1 (3.9208, -52.6617) -> (11.5814, -50.3565) centre (7.7511, -51.5091) ccw
  line L1 (11.5814, -50.3565) -> (10.3567, -46.2863)
  circle A2 centre (7.7511, -51.5091) radius 2.5
  circle A3 centre (7.7511, -51.5091) radius 1.5
  arc A4 (17.4138, 40.7753) -> (11.2138, 45.8311) centre (0, 25.75) ccw
  line L2 (17.4138, 40.7753) -> (20.1, 44.0694)
  arc A5 (20.1, 44.0694) -> (13.9, 49.1252) centre (17, 46.5973) ccw
  line L3 (13.9, 49.1252) -> (11.2138, 45.8311)
  circle A6 centre (17, 46.5973) radius 2.5
  circle A7 centre (17, 46.5973) radius 1.5
  dimension "d100" = 3
  constraint concentric A1 A3
  measures "d100" diameter of A3
extrude "Extrude7'" add sketch "Sketch20" along normal blind 2.25 contours A0 L0 A1 L1 | A2 | A4 L2 A5 L3 | A6 bodies 3 in component "Component"
copy_body "Body->Comp1" bodies 1 removing the originals makes body 5 in component "Mount"
split "Split1" [rolled back]
sketch "Sketch6" plane through (0, 0, 0) normal (0, 0, -1) x (-1, 0, 0)
  line L0 (-23, 13.25) -> (-18, 13.25)
  line L1 (-18, 13.25) -> (-18, -9.75)
  line L2 (-18, -9.75) -> (-23, -9.75)
  line L3 (-23, -9.75) -> (-23, -25.75)
  arc A0 (-23, -25.75) -> (23, -25.75) centre (0, -25.75) ccw
  line L4 (23, -25.75) -> (23, 25.75)
  arc A1 (23, 25.75) -> (-23, 25.75) centre (0, 25.75) ccw
  line L5 (-23, 25.75) -> (-23, 13.25)
  line L6 (-45.753, 76.4031) -> (79.6669, 76.4031)
  line L7 (79.6669, 76.4031) -> (79.6669, -77.5638)
  line L8 (79.6669, -77.5638) -> (-45.753, -77.5638)
  line L9 (-45.753, -77.5638) -> (-45.753, 76.4031)
  constraint horizontal L6
  constraint vertical L7
  constraint horizontal L8
  constraint vertical L9
extrude "Extrude8" [rolled back] along distance -14.7 taper angle 0
component "Component" placed x (1, 0, 0) y (0, 1, 0) z (0, 0, 1) at (0, 0, 0)
component "Mount" placed x (1, 0, 0) y (0, 1, 0) z (0, 0, 1) at (0, 0, 0)
hidden bodies 2
equation "d7 = 31 mm + 5 mm"
equation "d42 = 3.50 mm - 2.6 mm"
equation "d47 = 27.5 mm + ( 2 * 1.3 ) * 1 mm"
equation "d53 = -16.00 mm + 4.8 mm + 1.3 mm"
equation "d75 = -16.00 mm + 11.3 mm"
equation "d101 = -1.25 mm + 3.5 mm"
named bodies: "Projection"
